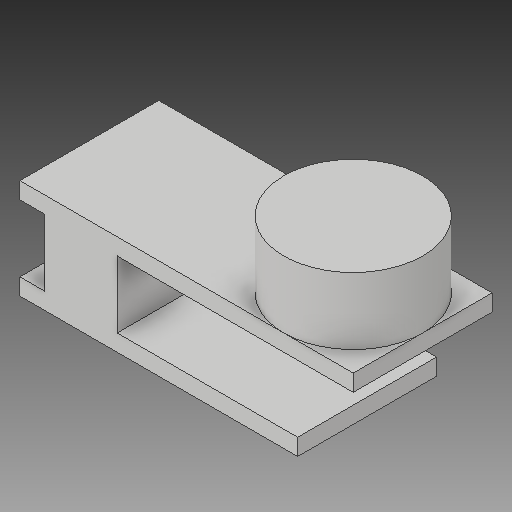
# Autodesk Inventor part: Lens
Saved by Autodesk Inventor 2017 (Build 210142000, 142)
## iProperties
Created: 2018-02-08
Part Number: Lens
Material: Generic
Document SubType Name: Modeling
Designer: Arjuna
Density: 1 g/cm^3
Appearance: Default
Author: Arjuna
Autodesk Inventor part; units mm, degrees
ref_plane "YZ Plane" through (0, 0, 0) normal (1, 0, 0) x (0, 1, 0)
ref_plane "XZ Plane" through (0, 0, 0) normal (0, 1, 0) x (-1, 0, 0)
ref_plane "XY Plane" through (0, 0, 0) normal (0, 0, 1) x (1, 0, 0)
sketch "Sketch6" plane through (0, 0, 0) normal (0, 0, 1) x (1, 0, 0)
  line L0 (-42.8333, 14.1784) -> (17.1667, 14.1784)
  line L1 (17.1667, 14.1784) -> (17.1667, 11.1784)
  line L2 (17.1667, 11.1784) -> (-42.8333, 11.1784)
  line L3 (-42.8333, 11.1784) -> (-42.8333, 14.1784)
  line L4 (-38.3333, 11.1784) -> (-25.3333, 11.1784)
  line L5 (-25.3333, 11.1784) -> (-25.3333, -0.8216)
  line L6 (-25.3333, -0.8216) -> (-38.3333, -0.8216)
  line L7 (-38.3333, -0.8216) -> (-38.3333, 11.1784)
  line L8 (-42.8333, -0.8216) -> (7.1667, -0.8216)
  line L9 (7.1667, -0.8216) -> (7.1667, -3.8216)
  line L10 (7.1667, -3.8216) -> (-42.8333, -3.8216)
  line L11 (-42.8333, -3.8216) -> (-42.8333, -0.8216)
  point P0 (0, 0)
  dimension "d27" = 3
  dimension "d28" = 60
  dimension "d29" = 13
  dimension "d30" = 4.5
  dimension "d31" = 12
  dimension "d34" = 50
  dimension "d35" = 3
  dimension "d36" = 0
  constraints: 24 end point, 6 parallel, 3 horizontal, 3 perpendicular, 1 point on line
  measures "d27" distance between parallel lines of L2 L0
  measures "d28" distance between parallel lines of L1 L3
  measures "d29" distance between parallel lines of L5 L7
  measures "d30" distance between parallel lines of L7 L3
  measures "d31" distance between parallel lines of L6 L2
  measures "d34" distance between parallel lines of L9 L11
  measures "d35" distance between parallel lines of L10 L8
  measures "d36" distance between parallel lines of L8 L6
extrude "Extrusion4" add sketch "Sketch6" along normal mid plane 25
sketch "Sketch7" plane through (-42.8333, 14.1784, 12.5) normal (0, 1, 0) x (1, 0, 0)
  circle A0 centre (47.5, 12.5) radius 12.5
  line L0 (60, 25) -> (60, 0) projected
  point P0 (42.8333, 12.5)
  dimension "d39" = 25
  dimension "d40" = 12.5
  constraints: 1 centre point
  measures "d39" diameter of A0
  measures "d40" distance from line of L0 A0.centre
extrude "Extrusion5" add sketch "Sketch7" along normal blind 12
equation "\"d40\" = 0.5 * d39"
body "Solid2"
